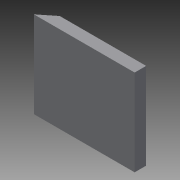
# Autodesk Inventor part: servo_clip2
Saved by Autodesk Inventor 2015 (Build 190159000, 159)
## iProperties
Created: 2017-12-02
Part Number: servo_clip2
Material: Generic
Document SubType Name: Modeling
Designer: Anshul
Density: 1 g/cm^3
Appearance: Default
Author: Anshul
Autodesk Inventor part; units mm, degrees
ref_plane "YZ Plane" through (0, 0, 0) normal (1, 0, 0) x (0, 1, 0)
ref_plane "XZ Plane" through (0, 0, 0) normal (0, 1, 0) x (-1, 0, 0)
ref_plane "XY Plane" through (0, 0, 0) normal (0, 0, 1) x (1, 0, 0)
sketch "Sketch1" plane through (0, 0, 0) normal (0, 1, 0) x (-1, 0, 0)
  line L0 (0, 0) -> (0, -16)
  line L1 (0, 0) -> (0, -30)
  line L2 (0, -16) -> (0, -20)
  line L3 (0, -16) -> (50, -16)
  line L4 (50, -16) -> (50, 0)
  line L5 (50, 0) -> (0, 0)
  line L6 (0, -20) -> (50, -20)
  line L7 (50, -20) -> (50, -16)
  line L8 (50, -20) -> (35, -20)
  line L9 (35, -20) -> (35, -22)
  line L10 (35, -22) -> (50, -22)
  line L11 (50, -22) -> (50, -20)
  line L12 (50, -22) -> (50, -27)
  line L13 (50, -27) -> (25, -27)
  line L14 (25, -27) -> (25, -20)
  line L15 (50, -20) -> (45, -20)
  line L16 (45, -20) -> (50, -16)
  line L17 (45, -20) -> (45, -22)
  line L18 (45, -22) -> (50, -27)
  line L19 (25, -27) -> (30, -27)
  line L20 (30, -27) -> (25, -20)
  line L21 (0, -16) -> (15, -16)
  line L22 (15, -16) -> (15, -20)
  dimension "d0" = 16
  dimension "d1" = 30
  dimension "d2" = 4
  dimension "d3" = 50
  dimension "d4" = 50
  dimension "d5" = 15
  dimension "d6" = 2
  dimension "d7" = 5
  dimension "d8" = 25
  dimension "d9" = 5
  dimension "d10" = 5
  dimension "d11" = 15
  constraints: 46 end point, 9 point on line, 8 perpendicular, 3 vertical, 1 midpoint
  measures "d0" distance of L0.start L0.end
  measures "d1" distance of L0.start L1.end
  measures "d2" distance of L0.end L2.end
  measures "d3" distance of L0.end L3.end
  measures "d4" distance of L2.end L6.end
  measures "d5" distance of L6.end L8.end
  measures "d6" distance of L8.end L9.end
  measures "d7" distance of L10.end L12.end
  measures "d8" distance of L12.end L13.end
  measures "d9" distance of L6.end L15.end
  measures "d10" distance of L13.end L19.end
  measures "d11" distance of L0.end L21.end
extrude "Extrusion1" add sketch "Sketch1" along normal blind 30 contours L3 L16 L6 L22
body "Solid1"
